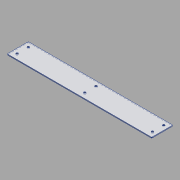
# Autodesk Inventor part: PBLMK-041-2
Saved by Autodesk Inventor 2016 (Build 200138000, 138)
## iProperties
Created: 2023-12-03
Part Number: PBLMK-041-2
Material: Aluminum
Document SubType Name: Modeling
Designer: Riskinova Oktavia
Density: 2.7 g/cm^3
Appearance: Aluminum - Flat
Description: LINEAR BRACKET
Author: Riskinova Oktavia
Autodesk Inventor part; units mm, degrees
ref_plane "YZ Plane" through (0, 0, 0) normal (1, 0, 0) x (0, 1, 0)
ref_plane "XZ Plane" through (0, 0, 0) normal (0, 1, 0) x (-1, 0, 0)
ref_plane "XY Plane" through (0, 0, 0) normal (0, 0, 1) x (1, 0, 0)
sketch "Sketch1" plane through (0, 0, 0) normal (0, 0, 1) x (1, 0, 0)
  line L0 (-240, 35) -> (240, 35)
  line L1 (240, 35) -> (240, -35)
  line L2 (240, -35) -> (-240, -35)
  line L3 (-240, -35) -> (-240, 35)
  line L4 (-240, 35) -> (240, -35) construction
  line L5 (240, 35) -> (-240, -35) construction
  point P0 (0, 0)
  dimension "d0" = 70
  dimension "d1" = 480
  constraints: 12 end point, 2 midpoint, 2 parallel, 1 horizontal, 1 perpendicular
  measures "d0" distance of L0.end L1.end
  measures "d1" distance of L0.start L0.end
extrude "Extrusion1" add sketch "Sketch1" along normal mid plane 3
sketch "Sketch2" plane through (0, 0, 1.5) normal (0, 0, 1) x (1, 0, 0)
  line L0 (-225.0001, 20) -> (225.0001, 20)
  line L1 (225.0001, 20) -> (225.0001, -17.5)
  line L2 (225.0001, -17.5) -> (-225.0001, -17.5)
  line L3 (-225.0001, -17.5) -> (-225.0001, 20)
  line L4 (240, 35) -> (-240, 35) projected
  line L5 (-240, -35) -> (240, -35) projected
  circle A0 centre (224.9999, -17.5) radius 2.3865 projected
  circle A1 centre (-225.0001, -17.5) radius 2.3865 projected
  point P0 (0, 0)
  point P1 (0, 20)
  point P2 (0, 20)
  point P3 (0, -17.5)
  dimension "d5" = 15
  constraints: 8 end point, 7 coincident, 2 midpoint, 2 parallel, 1 horizontal, 1 perpendicular, 1 vertical alignment
  measures "d5" distance from line of L0.start L4
hole "Hole1" at (-225.0001, 20, 1.5) at (-225.0001, -17.5, 1.5) at (225.0001, 20, 1.5) at (225.0001, -17.5, 1.5) at (0, 20, 1.5) at (0, -17.5, 1.5) direction (0, 0, -1) diameter 6.6 end through all
fillet "Fillet1" radius 2 4 edges at (240, -35, 0) (240, 35, 0) (-240, -35, 0) (-240, 35, 0)
body "Solid1"
